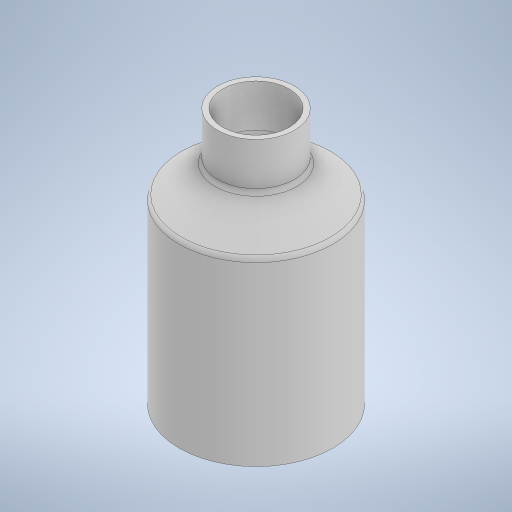
# Autodesk Inventor part: bottle
Saved by Autodesk Inventor 2024.2 (Build 282272000, 272)
## iProperties
Created: 2025-02-11
Part Number: bottle
Material: Generic
Document SubType Name: Modeling
Designer: Tom
Density: 1 g/cm^3
Appearance: Default
Author: Tom
Autodesk Inventor part; units mm, degrees
ref_plane "YZ Plane" through (0, 0, 0) normal (1, 0, 0) x (0, 1, 0)
ref_plane "XZ Plane" through (0, 0, 0) normal (0, 1, 0) x (-1, 0, 0)
ref_plane "XY Plane" through (0, 0, 0) normal (0, 0, 1) x (1, 0, 0)
sketch "Sketch1" plane through (0, 0, 0) normal (0, 0, 1) x (1, 0, 0)
  line L0 (0, 0) -> (0, 87.5741)
  line L1 (1.1889, 90.0512) -> (17.8611, 103.4187)
  line L2 (19.05, 105.8958) -> (19.05, 127)
  line L3 (19.05, 127) -> (38.1, 127)
  line L4 (38.1, 127) -> (38.1, 0)
  line L5 (38.1, 0) -> (0, 0)
  arc A0 (17.8611, 103.4187) -> (19.05, 105.8958) centre (15.875, 105.8958) ccw
  arc A1 (1.1889, 90.0512) -> (0, 87.5741) centre (3.175, 87.5741) ccw
  dimension "d0" = 127
  dimension "d1" = 38.1
  dimension "d2" = 19.05
  dimension "d3" = 3.175
  constraints: 12 end point, 4 point on circle, 4 tangent, 3 perpendicular, 2 centre point, 1 equal radius, 1 parallel, 1 vertical
  measures "d0" distance of L3.end L4.end
  measures "d1" distance of L4.end L0.start
  measures "d2" distance of L2.end L3.end
  measures "d3" radius of A0
revolve "Revolution1" add sketch "Sketch1" angle 360 about axis through (38.1, 127, 0) along (0, -1, 0)
shell "Shell1" thickness 2.54 removed faces 1 at (38.9963, 127, 5.2259)
body "Solid1"
